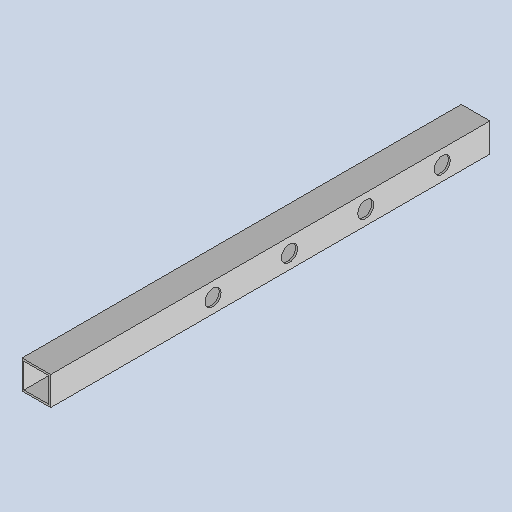
# Autodesk Inventor part: PRS 1662 DrSysB way tube 2_1200
Saved by Autodesk Inventor 2026.2 (Build 302298000, 298)
## iProperties
Created: 2025-06-24
Part Number: PRS 1662 DrSysB way tube 2_1200
Material: Stainless Steel
Document SubType Name: Modeling
Designer: admin
Mass: 1762.25 g
Surface Area: 2283.33 cm^2
Volume: 220.281 cm^3
Density: 8 g/cm^3
Sheet Metal Rule: AISI304 2mm Die16
Sheet Metal Width: 0.000 mm
Sheet Metal Length: 0.000 mm
Sheet Metal Area: 0.000 mm^2
Appearance: Default
Author: user
Autodesk Inventor part; units mm, degrees
ref_plane "YZ Plane" through (0, 0, 0) normal (1, 0, 0) x (0, 1, 0)
ref_plane "XZ Plane" through (0, 0, 0) normal (0, 1, 0) x (-1, 0, 0)
ref_plane "XY Plane" through (0, 0, 0) normal (0, 0, 1) x (1, 0, 0)
sketch "Sketch9" plane through (0, 0, 0) normal (0, 1, 0) x (-1, 0, 0)
  line L0 (15, 15) -> (-15, 15)
  line L1 (-15, 15) -> (-15, -15)
  line L2 (-15, -15) -> (15, -15)
  line L3 (15, -15) -> (15, 15)
  line L4 (15, 15) -> (-15, -15) construction
  line L5 (-15, 15) -> (15, -15) construction
  line L6 (-13, 13) -> (13, 13)
  line L7 (13, 13) -> (13, -13)
  line L8 (13, -13) -> (-13, -13)
  line L9 (-13, -13) -> (-13, 13)
  point P0 (0, 0)
  dimension "d172" = 30
  dimension "d173" = 30
  dimension "d174" = 2
  constraints: 20 end point, 4 parallel, 2 midpoint, 2 perpendicular, 1 horizontal, 3 other
  measures "d172" distance of L2.end L1.end
  measures "d173" distance of L0.end L1.end
  measures "d174" distance between parallel lines of L0 L6
extrude "Extrusion3" add sketch "Sketch9" against normal blind 460
sketch "Sketch10" plane through (0, 0, 0) normal (1, 0, 0) x (0, 1, 0)
  line L0 (0, 15) -> (0, -15) construction
  line L1 (0, 15) -> (-460, 15) construction
  line L2 (0, -15) -> (-460, -15) construction
  line L3 (-58.5, 8.5) -> (-41.5, 8.5)
  line L4 (-41.5, 8.5) -> (-41.5, -8.5)
  line L5 (-41.5, -8.5) -> (-58.5, -8.5)
  line L6 (-58.5, -8.5) -> (-58.5, 8.5)
  line L7 (-58.5, 8.5) -> (-41.5, -8.5) construction
  line L8 (-41.5, 8.5) -> (-58.5, -8.5) construction
  line L9 (0, 0) -> (30, 0)
  circle A0 centre (-50, 0) radius 8.5
  dimension "d177" = 17
  dimension "d178" = 17
  dimension "d181" = 30
  dimension "d182" = 80
  constraints: 14 end point, 3 midpoint, 2 horizontal, 2 parallel, 1 centre point, 1 coincident, 1 horizontal alignment, 1 perpendicular, 1 tangent
  measures "d177" distance of L3.start L3.end
  measures "d178" distance of L3.end L4.end
  measures "d181" distance of L9.start L9.end
  measures "d182" distance of point (-50, 0) L9.end
extrude "Extrusion4" cut sketch "Sketch10" along normal through all contours A0
pattern_linear "Rectangular Pattern4" count 4 spacing 80 along (0, -1, 0) of "Extrusion4"
body "Solid4"
